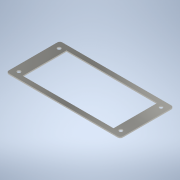
# Autodesk Inventor part: metal_holder
Saved by Autodesk Inventor 2022 (Build 260153000, 153)
## iProperties
Created: 2022-07-20
Part Number: metal_holder
Material: Серебро
Document SubType Name: Modeling
Designer: akapu
Density: 10.49 g/cm^3
Appearance: Серебро
Author: akapu
Autodesk Inventor part; units mm, degrees
ref_plane "YZ Plane" through (0, 0, 0) normal (1, 0, 0) x (0, 1, 0)
ref_plane "XZ Plane" through (0, 0, 0) normal (0, 1, 0) x (-1, 0, 0)
ref_plane "XY Plane" through (0, 0, 0) normal (0, 0, 1) x (1, 0, 0)
sketch "Эскиз1" plane through (0, 0, 0) normal (0, 1, 0) x (-1, 0, 0)
  line L0 (0, 0) -> (75.2, 0)
  line L1 (75.2, 0) -> (75.2, 36.7)
  line L2 (75.2, 36.7) -> (0, 36.7)
  line L3 (0, 36.7) -> (0, 0)
  line L4 (0, 0) -> (-10, 0)
  line L5 (-10, 0) -> (-10, -4)
  line L6 (-10, -4) -> (0, -4)
  line L7 (0, -4) -> (0, 0)
  line L8 (-10, -4) -> (85.2, -4)
  line L9 (85.2, -4) -> (85.2, 40.7)
  line L10 (85.2, 40.7) -> (-10, 40.7)
  line L11 (-10, 40.7) -> (-10, -4)
  line L12 (75.2, 36.7) -> (80.2, 36.7)
  line L13 (80.2, 36.7) -> (80.2, 0)
  line L14 (80.2, 0) -> (80.2, 36.7)
  line L15 (80.2, 36.7) -> (80.2, 35.15)
  line L16 (80.2, 0) -> (80.2, 1.55)
  line L17 (0, 0) -> (-5, 0)
  line L18 (-5, 0) -> (-5, 1.55)
  line L19 (-5, 1.55) -> (-5, 36.7)
  line L20 (-5, 36.7) -> (-5, 35.15)
  circle A0 centre (-5, 35.15) radius 1.5
  circle A1 centre (-5, 1.55) radius 1.5
  circle A2 centre (80.2, 35.15) radius 1.5
  circle A3 centre (80.2, 1.55) radius 1.5
  dimension "d0" = 75.2
  dimension "d1" = 36.7
  dimension "d2" = 10
  dimension "d3" = 4
  dimension "d4" = 95.2
  dimension "d5" = 44.7
  dimension "d6" = 5
  dimension "d7" = 1.55
  dimension "d8" = 1.55
  dimension "d9" = 5
  dimension "d10" = 1.55
  dimension "d11" = 1.55
  dimension "d12" = 3
  dimension "d13" = 3
  dimension "d14" = 3
  dimension "d15" = 3
  constraints: 42 end point, 7 equal length, 6 perpendicular, 4 centre point, 4 coincident, 4 point on line, 3 horizontal, 1 midpoint
  measures "d0" distance of L2.end L1.end
  measures "d1" distance of L1.end L0.end
  measures "d2" distance of L6.end L5.end
  measures "d3" distance of L5.end L4.end
  measures "d4" distance of L10.end L9.end
  measures "d5" distance of L9.end L8.end
  measures "d6" distance of L1.end L12.end
  measures "d7" distance of L12.end L15.end
  measures "d8" distance of L13.end L16.end
  measures "d9" distance of L0.start L17.end
  measures "d10" distance of L17.end L18.end
  measures "d11" distance of L19.end L20.end
  measures "d12" diameter of A0
  measures "d13" diameter of A1
  measures "d14" diameter of A2
  measures "d15" diameter of A3
extrude "Выдавливание1" add sketch "Эскиз1" along normal blind 1
fillet "Сопряжение1" radius 2 4 edges at (-85.2, 0.5, 40.7) (-85.2, 0.5, -4) (10, 0.5, -4) (10, 0.5, 40.7)
sketch "Эскиз2" plane through (0, 1, 0) normal (0, 1, 0) x (1, 0, 0)
  line L0 (0, 0) -> (0.4, 0)
  line L1 (0.4, 0) -> (-75.6, 0)
  line L2 (-75.6, 0) -> (-75.6, -36.7)
  line L3 (-75.6, -36.7) -> (0.4, -36.7)
  line L4 (0.4, -36.7) -> (0.4, 0)
  dimension "d19" = 0.4
  dimension "d20" = 76
  constraints: 10 end point, 2 horizontal, 2 parallel, 1 perpendicular
  measures "d19" distance of L0.start L0.end
  measures "d20" distance of L3.end L2.end
extrude "Выдавливание2" cut sketch "Эскиз2" against normal blind 10
